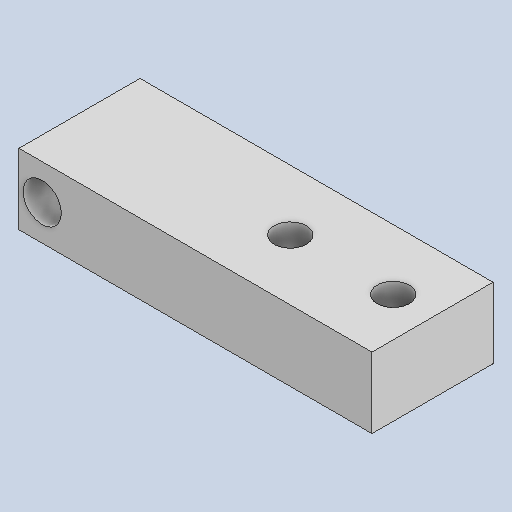
# Autodesk Inventor part: dedos
Saved by Autodesk Inventor 2024.3 (Build 283343000, 343)
## iProperties
Created: 2025-07-08
Part Number: dedos
Material: Generic
Document SubType Name: Modeling
Designer: user
Density: 1 g/cm^3
Appearance: Default
Author: user
Autodesk Inventor part; units mm, degrees
ref_plane "YZ Plane" through (0, 0, 0) normal (1, 0, 0) x (0, 1, 0)
ref_plane "XZ Plane" through (0, 0, 0) normal (0, 1, 0) x (-1, 0, 0)
ref_plane "XY Plane" through (0, 0, 0) normal (0, 0, 1) x (1, 0, 0)
sketch "Sketch1" plane through (0, 0, 0) normal (0, 0, 1) x (1, 0, 0)
  circle A0 centre (8.4, -37.55) radius 1.9 projected
  circle A1 centre (8.4, -7.35) radius 1.9 projected
  line L0 (19, -44.9) -> (0, -44.9) projected
  line L1 (19, 0) -> (19, -44.9) projected
  line L2 (0, 0) -> (19, 0) projected
  line L3 (0, 0) -> (0, -44.9) projected
  line L4 (41.1, -3.85) -> (6.1, -3.85)
  line L5 (6.1, -3.85) -> (6.1, -10.85)
  line L6 (6.1, -10.85) -> (41.1, -10.85)
  line L7 (41.1, -10.85) -> (41.1, -3.85)
  point P0 (41, -7.35)
  point P1 (30.9, -7.35)
  dimension "d0" = 35
  dimension "d1" = 7
  constraints: 8 end point, 2 parallel, 1 horizontal, 1 perpendicular
  measures "d0" distance of L6.end L5.end
  measures "d1" distance of L5.end L4.end
extrude "Extrusion1" add sketch "Sketch1" along normal blind 12 contours L6 L5 L4 L1 | L1 L4 L7 L6
sketch "Sketch2" plane through (6.1, -3.85, 0) normal (0, 1, 0) x (1, 0, 0)
  line L0 (35, 0) -> (0, 0) projected
  line L1 (0, 0) -> (0, -12) projected
  line L2 (35, -12) -> (0, -12) projected
  line L3 (35, 0) -> (35, -12) projected
  line L4 (35, -6) -> (0, -6)
  circle A0 centre (20.9, -6) radius 1.6
  line L5 (19.3, -6) -> (32.7, -6)
  line L6 (32.7, -6) -> (31.1, -6)
  circle A1 centre (31.1, -6) radius 1.6
  line L7 (32.7, -6) -> (35, -6)
  point P0 (-6.1, 0)
  dimension "d5" = 3.2
  dimension "d6" = 13.4
  dimension "d7" = 1.6
  dimension "d8" = 2.3
  constraints: 8 end point, 4 point on line, 3 coincident, 2 centre point, 2 midpoint
  measures "d5" diameter of A0
  measures "d6" distance of L5.start L5.end
  measures "d7" distance of L5.end L6.end
  measures "d8" distance of L5.end L7.end
extrude "Extrusion2" cut sketch "Sketch2" against normal blind 12 contours A1 L4 | L4 A1 | A0 L4 | L4 A0
body "Solid1"
